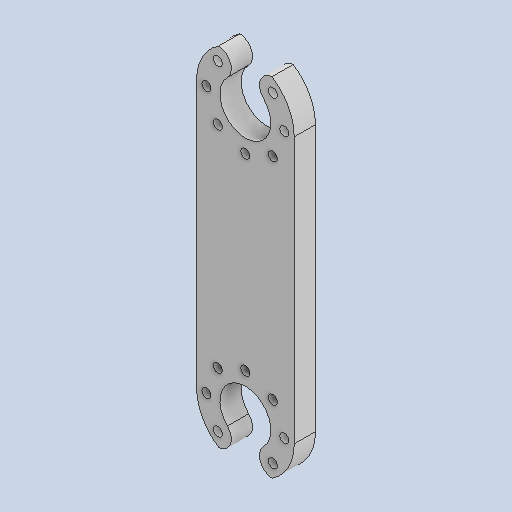
# Autodesk Inventor part: _shim
Saved by Autodesk Inventor 2024.3 (Build 283343000, 343)
## iProperties
Created: 2024-09-05
Part Number: _shim
Material: 일반
Document SubType Name: Modeling
Designer: gretc
Density: 1 g/cm^3
Appearance: 기본값
Author: gretc
Autodesk Inventor part; units mm, degrees
ref_plane "YZ Plane" through (0, 0, 0) normal (1, 0, 0) x (0, 1, 0)
ref_plane "XZ Plane" through (0, 0, 0) normal (0, 1, 0) x (-1, 0, 0)
ref_plane "XY Plane" through (0, 0, 0) normal (0, 0, 1) x (1, 0, 0)
sketch "스케치1" plane through (0, 0, 0) normal (0, 0, 1) x (1, 0, 0)
  circle A0 centre (0, 0) radius 13.8 projected
  circle A1 centre (0, 0) radius 7.2 projected
  circle A2 centre (0, -11) radius 1.2812 projected
  circle A3 centre (-7.7782, -7.7782) radius 1.2812 projected
  circle A4 centre (-11, 0) radius 1.2812 projected
  circle A5 centre (-7.7782, 7.7782) radius 1.2812 projected
  circle A6 centre (0, 11) radius 1.2812 projected
  circle A7 centre (7.7782, 7.7782) radius 1.2812 projected
  circle A8 centre (11, 0) radius 1.2812 projected
  circle A9 centre (7.7782, -7.7782) radius 1.2812 projected
  circle A10 centre (0, 75.1) radius 13.8 projected
  circle A11 centre (0, 75.1) radius 7.2 projected
  circle A12 centre (0, 64.1) radius 1.2812 projected
  circle A13 centre (-7.7782, 67.3218) radius 1.2812 projected
  circle A14 centre (-11, 75.1) radius 1.2812 projected
  circle A15 centre (-7.7782, 82.8782) radius 1.2812 projected
  circle A16 centre (0, 86.1) radius 1.2812 projected
  circle A17 centre (7.7782, 82.8782) radius 1.2812 projected
  circle A18 centre (11, 75.1) radius 1.2812 projected
  circle A19 centre (7.7782, 67.3218) radius 1.2812 projected
  circle A20 centre (7.7782, -7.7782) radius 3.8
  circle A21 centre (-7.7782, -7.7782) radius 3.8
  line L0 (-113.808, 75.1) -> (55.228, 75.1)
  line L1 (13.8, 0) -> (13.8, 75.1)
  line L2 (-13.8, 0) -> (-13.8, 75.1)
  circle A22 centre (7.7782, 82.8782) radius 3.8
  circle A23 centre (-7.7782, 82.8782) radius 3.8
  point P0 (0, 0)
  point P1 (5.0912, -5.0912)
  point P2 (7.5223, -11.5696)
  point P3 (7.5223, 86.6696)
  point P4 (5.0912, 80.1912)
  point P5 (-5.0912, 80.1912)
  point P6 (-7.5223, 86.6696)
  point P7 (-7.5223, -11.5696)
  point P8 (-5.0912, -5.0912)
  constraints: 6 end point, 5 tangent, 4 centre point, 4 coincident, 4 point on circle, 2 point on line, 1 horizontal, 1 parallel, 1 vertical, 2 other
extrude "돌출1" add sketch "스케치1" along normal blind 6 contours A0 A20 A1 A21 | A0 L2 A10 L1 | A0 A20 | L0 A18 A11 A22 A10 | A10 L0 A14 A11 A18 | A21 A0 | A10 A23 A11 L0 A14 | A22 A10 | A10 A23 picked at (4.2604, 10.6567) picked at (10.3474, -8.1187) picked at (-10.3474, -8.1187) picked at (10.3474, 83.2187) picked at (-10.3474, 83.2187)
